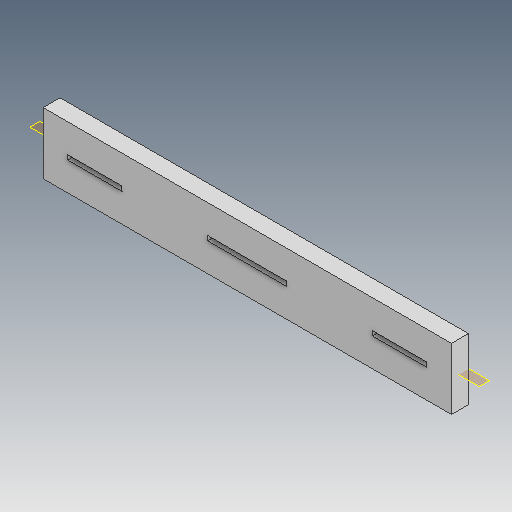
# Autodesk Inventor part: mid_bottom
Saved by Autodesk Inventor 2020 (Build 240168000, 168)
## iProperties
Created: 2021-05-08
Part Number: mid_bottom
Material: Generic
Document SubType Name: Modeling
Designer: Hsu Daniel
Density: 1 g/cm^3
Appearance: Default
Author: Hsu Daniel
Autodesk Inventor part; units mm, degrees
ref_plane "YZ Plane" through (0, 0, 0) normal (1, 0, 0) x (0, 1, 0)
ref_plane "XZ Plane" through (0, 0, 0) normal (0, 1, 0) x (-1, 0, 0)
sketch "Sketch1" plane through (0, 0, 0) normal (0, 0, 1) x (1, 0, 0)
  line L0 (0, 0) -> (132.6, 0)
  line L1 (132.6, 0) -> (132.6, 20)
  line L2 (132.6, 20) -> (0, 20)
  line L3 (0, 20) -> (0, 0)
  line L4 (0, 10) -> (132.6, 10) construction
  line L5 (66.3, 20) -> (66.3, 0) construction
  line L6 (53.45, 9.25) -> (79.15, 9.25)
  line L7 (79.15, 9.25) -> (79.15, 10.75)
  line L8 (79.15, 10.75) -> (53.45, 10.75)
  line L9 (53.45, 10.75) -> (53.45, 9.25)
  line L10 (53.45, 9.25) -> (79.15, 10.75) construction
  line L11 (79.15, 9.25) -> (53.45, 10.75) construction
  line L12 (8, 9.25) -> (25.6, 9.25)
  line L13 (25.6, 9.25) -> (25.6, 10.75)
  line L14 (25.6, 10.75) -> (8, 10.75)
  line L15 (8, 10.75) -> (8, 9.25)
  line L16 (8, 9.25) -> (25.6, 10.75) construction
  line L17 (25.6, 9.25) -> (8, 10.75) construction
  line L18 (107, 9.25) -> (124.6, 9.25)
  line L19 (124.6, 9.25) -> (124.6, 10.75)
  line L20 (124.6, 10.75) -> (107, 10.75)
  line L21 (107, 10.75) -> (107, 9.25)
  line L22 (107, 9.25) -> (124.6, 10.75) construction
  line L23 (124.6, 9.25) -> (107, 10.75) construction
  point P0 (66.3, 10)
  point P1 (16.8, 10)
  point P2 (115.8, 10)
  dimension "d0" = 132.6
  dimension "d1" = 20
  dimension "d2" = 25.7
  dimension "d3" = 1.5
  dimension "d4" = 17.6
  dimension "d5" = 1.5
  dimension "d6" = 49.5
  dimension "d7" = 17.6
  dimension "d8" = 1.5
  dimension "d9" = 49.5
  constraints: 48 end point, 11 midpoint, 8 parallel, 4 horizontal, 4 perpendicular, 2 point on line
  measures "d0" distance of L2.end L1.end
  measures "d1" distance of L1.end L0.end
  measures "d2" distance of L8.end L7.end
  measures "d3" distance of L6.end L7.end
  measures "d4" distance of L14.end L13.end
  measures "d5" distance of L12.end L13.end
  measures "d6" distance of point (66.3, 10) point (16.8, 10)
  measures "d7" distance of L19.end L20.end
  measures "d8" distance of L18.end L19.end
  measures "d9" distance of point (66.3, 10) point (115.8, 10)
extrude "Extrusion1" add sketch "Sketch1" along normal blind 5.5
ref_plane "Work Plane1" through (0, 10, 0) normal (0, 1, 0) x (1, 0, 0)
ref_plane "Work Plane2" through (66.3, 0, 0) normal (1, 0, 0) x (0, 0, -1)
equation "\"d1\" = midbottomw"
equation "\"d2\" = mmid + toler"
equation "\"d4\" = mlr + toler"
equation "\"d5\" = d3"
equation "\"d6\" = mbetween"
equation "\"d7\" = d4"
equation "\"d8\" = d3"
equation "\"d9\" = d6"
equation "\"thick\" = 0.5"
equation "\"lrlr\" = 19"
equation "\"lrmid\" = 19.9"
equation "\"lrdepth\" = 3.3"
equation "\"mlr\" = 16.6"
equation "\"mmid\" = 24.7"
equation "\"mdepth\" = 4.5"
equation "\"lrltotal\" = 126.6"
equation "\"mltotal\" = 126.6"
equation "\"lrbetween\" = 52.1"
equation "\"mbetween\" = 49.5"
equation "\"toler\" = 1"
equation "\"midbottomw\" = 20"
equation "\"stuckw\" = 6"
equation "\"tight\" = 0.08"
equation "\"sidewallL\" = 132.6"
equation "\"heaterH\" = 117.3"
equation "\"stickL\" = 3.5"
equation "\"wireH\" = 25"
body "Solid1"
